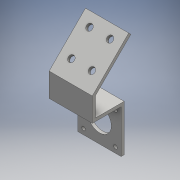
# Autodesk Inventor part: 电机座1
Saved by Autodesk Inventor 2016 (Build 200138000, 138)
## iProperties
Created: 2019-04-02
Part Number: 电机座1
Material: 常规
Document SubType Name: Modeling
Designer: oldboy
Density: 1 g/cm^3
Appearance: 默认
Author: oldboy
Autodesk Inventor part; units mm, degrees
ref_plane "YZ Plane" through (0, 0, 0) normal (1, 0, 0) x (0, 1, 0)
ref_plane "XZ Plane" through (0, 0, 0) normal (0, 1, 0) x (-1, 0, 0)
sketch "草图2" plane through (0, 0, 0) normal (0, 1, 0) x (-1, 0, 0)
  line L0 (-21, 21) -> (21, 21)
  line L1 (21, 21) -> (21, -21)
  line L2 (21, -21) -> (-21, -21)
  line L3 (-21, -21) -> (-21, 21)
  line L4 (-21, 21) -> (21, -21) construction
  line L5 (21, 21) -> (-21, -21) construction
  point P0 (0, 0)
  dimension "d3" = 42
  dimension "d4" = 42
  constraints: 12 end point, 2 midpoint, 2 parallel, 1 horizontal, 1 perpendicular
  measures "d3" distance between parallel lines of L3 L1
  measures "d4" distance between parallel lines of L2 L0
extrude "拉伸2" add sketch "草图2" along normal blind 3
sketch "草图3" plane through (-21, 0, 21) normal (0, 0, 1) x (1, 0, 0)
  line L0 (0, 3) -> (42, 3) projected
  line L1 (0, 3) -> (42, 3)
  line L2 (42, 3) -> (42, -48)
  line L3 (42, -48) -> (0, -48)
  line L4 (0, -48) -> (0, 3)
  point P0 (21, 0)
  dimension "d7" = 51
  constraints: 8 end point, 2 parallel, 1 horizontal, 1 perpendicular
  measures "d7" distance between parallel lines of L3 L0
extrude "拉伸3" add sketch "草图3" along normal blind 3
ref_plane "工作平面1" through (-21, -48, 24) normal (0, -0.7071, 0.7071) x (1, 0, 0)
sketch "草图7" plane through (0, 0, 0) normal (0, -1, 0) x (1, 0, 0)
  circle A0 centre (0, 0) radius 11.5
  circle A1 centre (-15.5, 15.5) radius 1.75
  circle A2 centre (-15.5, -15.5) radius 1.75
  circle A3 centre (15.5, -15.5) radius 1.75
  circle A4 centre (15.5, 15.5) radius 1.75
  dimension "d17" = 23
  dimension "d18" = 3.5
  dimension "d19" = 15.5
  dimension "d20" = 15.5
  dimension "d21" = 15.5
  dimension "d22" = 15.5
  constraints: 5 centre point, 3 equal radius, 2 horizontal alignment, 2 vertical alignment, 1 coincident
  measures "d17" diameter of A0
  measures "d18" diameter of A2
  measures "d19" horizontal distance of point (0, 0) A2.centre
  measures "d20" horizontal distance of point (0, 0) A2.centre
  measures "d21" horizontal distance of point (0, 0) A1.centre
  measures "d22" horizontal distance of point (0, 0) A3.centre
extrude "拉伸6" cut sketch "草图7" against normal blind 3
sketch "草图9" plane through (-21, 0, 24) normal (0, 0, 1) x (1, 0, 0)
  line L0 (0, 0) -> (0, -48) projected
  line L1 (42, -48) -> (42, 0) projected
  line L2 (0, -28) -> (42, -28)
  line L3 (42, -28) -> (42, -25)
  line L4 (42, -25) -> (0, -25)
  line L5 (0, -25) -> (0, -28)
  line L6 (0, -48) -> (42, -48) projected
  point P0 (21, 0)
  dimension "d32" = 3
  dimension "d33" = 20
  constraints: 8 end point, 2 parallel, 2 point on line, 1 horizontal, 1 perpendicular
  measures "d32" distance between parallel lines of L2 L4
  measures "d33" distance between parallel lines of L6 L2
extrude "拉伸8" add sketch "草图9" along normal blind 20 contours L4 L1 L2 L0
sketch "草图10" plane through (-21, 0, 24) normal (0, 0, 1) x (1, 0, 0)
  line L0 (42, -28) -> (0, -28) projected
  line L1 (0, -28) -> (0, -48) projected
  line L2 (0, -48) -> (42, -48) projected
  line L3 (42, -48) -> (42, -28) projected
  point P0 (21, 0)
extrude "拉伸9" cut sketch "草图10" against normal blind 20
sketch "草图11" plane through (-21, -48, 24) normal (0, -0.7071, 0.7071) x (1, 0, 0)
  line L0 (0, 28.2843) -> (42, 28.2843) projected
  line L1 (0, 28.2843) -> (42, 28.2843)
  line L2 (42, 28.2843) -> (42, 78.2843)
  line L3 (42, 78.2843) -> (0, 78.2843)
  line L4 (0, 78.2843) -> (0, 28.2843)
  point P0 (21, 16.9706)
  dimension "d38" = 42
  dimension "d39" = 50
  constraints: 8 end point, 2 parallel, 1 horizontal, 1 perpendicular
  measures "d38" distance between parallel lines of L2 L4
  measures "d39" distance between parallel lines of L0 L3
extrude "拉伸10" add sketch "草图11" against normal blind 3
sketch "草图12" plane through (-21, -48, 24) normal (0, -0.7071, 0.7071) x (1, 0, 0)
  line L0 (0, 28.2843) -> (42, 28.2843) construction
  line L1 (21, 28.2843) -> (21, 78.2843) construction
  line L2 (0, 78.2843) -> (42, 78.2843) construction
  circle A0 centre (31, 43.2843) radius 3
  circle A1 centre (31, 68.2843) radius 3
  circle A2 centre (11, 43.2843) radius 3
  circle A3 centre (11, 68.2843) radius 3
  point P0 (21, 16.9706)
  dimension "d42" = 6
  dimension "d43" = 10
  dimension "d44" = 15
  dimension "d45" = 25
  constraints: 4 centre point, 2 end point, 2 midpoint, 2 symmetric about line, 1 equal radius, 1 vertical alignment, 2 other
  measures "d42" diameter of A0
  measures "d43" distance from line of L1 A0.centre
  measures "d44" distance from line of L0 A0.centre
  measures "d45" distance of A1.centre A0.centre
extrude "拉伸11" cut sketch "草图12" against normal blind 3
